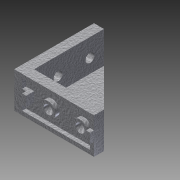
# Autodesk Inventor part: Corner Brace
Saved by Autodesk Inventor 2015 SP1 (Build 190203100, 203)
## iProperties
Created: 2015-03-03
Part Number: Corner Brace
Material: Aluminum 6061
Document SubType Name: Modeling
Designer: Andrew
Density: 2.7 g/cm^3
Appearance: Aluminum Cast
Author: Andrew
Autodesk Inventor part; units mm, degrees
ref_plane "YZ Plane" through (0, 0, 0) normal (1, 0, 0) x (0, 1, 0)
ref_plane "XZ Plane" through (0, 0, 0) normal (0, 1, 0) x (-1, 0, 0)
ref_plane "XY Plane" through (0, 0, 0) normal (0, 0, 1) x (1, 0, 0)
sketch "Sketch1" plane through (0, 0, 0) normal (0, 0, 1) x (1, 0, 0)
  line L0 (0, 0) -> (0, 35)
  line L1 (0, 35) -> (-3, 35)
  line L2 (-3, 35) -> (-3, -3)
  line L3 (-3, -3) -> (35, -3)
  line L4 (35, -3) -> (35, 0)
  line L5 (35, 0) -> (0, 0)
  line L6 (0, 35) -> (35, 0)
  dimension "d0" = 38
  dimension "d1" = 3
  constraints: 14 end point, 7 perpendicular, 1 vertical
  measures "d0" distance between parallel lines of L4 L2
  measures "d1" distance of L0.end L1.end
extrude "Extrusion1" add sketch "Sketch1" along normal blind 18 contours L5 L4 L3 L2 L1 L0
extrude "Extrusion2" add sketch "Sketch1" along normal blind 2 contours L0 L6 L5
sketch "Sketch2" plane through (-3, -3, 0) normal (-1, 0, 0) x (0, 0, 1)
  line L0 (0, 38) -> (0, 0) projected
  line L1 (0, 0) -> (18, 0) projected
  line L2 (18, 38) -> (18, 0) projected
  line L3 (0, 38) -> (18, 38) projected
  line L4 (16, 36) -> (2, 36)
  line L5 (2, 36) -> (2, 2)
  line L6 (2, 2) -> (6.5, 2)
  line L7 (6.5, 2) -> (6.5, 6)
  line L8 (6.5, 6) -> (11.5, 6)
  line L9 (11.5, 6) -> (11.5, 2)
  line L10 (11.5, 2) -> (16, 2)
  line L11 (16, 2) -> (16, 36)
  line L12 (9, 6) -> (9, 0) construction
  line L13 (6.5, 4) -> (11.5, 4)
  line L14 (0, 38) -> (18, 38) projected
  line L15 (6.5, 38) -> (6.5, 36)
  line L16 (11.5, 36) -> (11.5, 38)
  circle A0 centre (9, 31) radius 3.75
  circle A1 centre (9, 15) radius 3.75
  circle A2 centre (9, 31) radius 2.25
  circle A3 centre (9, 15) radius 2.25
  circle A4 centre (9, 31) radius 3
  circle A5 centre (9, 15) radius 3
  line L17 (9, 38) -> (9, 6) construction
  point P0 (0, 3)
  dimension "d6" = 2
  dimension "d7" = 2
  dimension "d8" = 2
  dimension "d9" = 2
  dimension "d10" = 5
  dimension "d11" = 4
  dimension "d12" = 4.5
  dimension "d13" = 0.75
  dimension "d14" = 0.75
  dimension "d15" = 16
  dimension "d16" = 5
  constraints: 26 end point, 8 point on line, 7 perpendicular, 6 centre point, 5 midpoint, 4 coincident, 3 equal radius, 2 collinear, 1 horizontal, 1 parallel, 1 vertical, 1 other
  measures "d6" distance between parallel lines of L0 L5
  measures "d7" distance between parallel lines of L3 L4
  measures "d8" distance between parallel lines of L2 L11
  measures "d9" distance between parallel lines of L1 L6
  measures "d10" distance between parallel lines of L9 L7
  measures "d11" distance between parallel lines of L10 L8
  measures "d12" diameter of A2
  measures "d13" radial gap between concentric circles of A4 A2
  measures "d14" radial gap between concentric circles of A0 A4
  measures "d15" distance of A0.centre A1.centre
  measures "d16" distance from line of L4 A0.centre
extrude "Extrusion3" add sketch "Sketch2" along normal blind 2 contours L3 L15 L4 L5 L6 L7 L13 L9 L10 L11 L16 L2 L1 L0 | L3 L16 L4 L15
extrude "Extrusion4" add sketch "Sketch2" along normal blind 4 contours L3 L16 L4 L15
extrude "Extrusion5" add sketch "Sketch2" along normal blind 4 contours L7 L8 L9 L13
extrude "Extrusion6" add sketch "Sketch2" along normal up to surface (2 mm away) contours A0 | A1 | A4 | A5
extrude "Extrusion7" cut sketch "Sketch2" against normal up to next contours A2 | A3
chamfer "Chamfer1" distance 2 angle 15 1 edges at (-5, 28, 5.25) measured on face at (-4.5, 28, 5.25)
chamfer "Chamfer2" distance 2 angle 15 1 edges at (-5, 12, 5.25) measured on face at (-4.5, 12, 5.25)
sketch "Sketch3" plane through (35, -3, 0) normal (0, -1, 0) x (1, 0, 0)
  line L0 (-2, 16) -> (-2, 2)
  line L1 (-2, 2) -> (-36, 2)
  line L2 (-36, 2) -> (-36, 11.5)
  line L3 (-36, 11.5) -> (-32, 11.5)
  line L4 (-32, 11.5) -> (-32, 6.5)
  line L5 (-32, 6.5) -> (-36, 6.5)
  line L6 (-36, 6.5) -> (-36, 16)
  line L7 (-36, 16) -> (-2, 16)
  line L8 (-32, 9) -> (-40, 9) construction
  line L9 (-34, 11.5) -> (-34, 6.5)
  line L10 (0, 11.5) -> (-2, 11.5)
  line L11 (-2, 6.5) -> (0, 6.5)
  circle A0 centre (-7, 9) radius 3.75
  circle A1 centre (-23, 9) radius 3.75
  circle A2 centre (-7, 9) radius 2.25
  circle A3 centre (-23, 9) radius 2.25
  circle A4 centre (-7, 9) radius 3
  circle A5 centre (-23, 9) radius 3
  line L12 (0, 9) -> (-32, 9) construction
  line L13 (0, 0) -> (-40, 0) projected
  line L14 (0, 0) -> (0, 18) projected
  line L15 (0, 18) -> (-40, 18) projected
  line L16 (-40, 0) -> (-40, 18) projected
  line L17 (0, 0) -> (0, 18) projected
  point P0 (-35, 0)
  point P1 (0, 3)
  dimension "d37" = 5
  dimension "d38" = 4
  dimension "d39" = 4.5
  dimension "d40" = 0.75
  dimension "d41" = 0.75
  dimension "d42" = 16
  dimension "d43" = 5
  dimension "d44" = 2
  dimension "d45" = 4
  dimension "d46" = 2
  constraints: 26 end point, 8 point on line, 6 centre point, 6 perpendicular, 5 midpoint, 4 coincident, 3 collinear, 3 equal radius, 1 parallel, 1 other
  measures "d37" distance between parallel lines of L5 L3
  measures "d38" distance between parallel lines of L6 L4
  measures "d39" diameter of A2
  measures "d40" radial gap between concentric circles of A4 A2
  measures "d41" radial gap between concentric circles of A0 A4
  measures "d42" distance of A0.centre A1.centre
  measures "d43" distance from line of L0 A0.centre
  measures "d44" distance between parallel lines of L13 L1
  measures "d45" distance between parallel lines of L16 L2
  measures "d46" distance between parallel lines of L14 L0
extrude "Extrusion8" add sketch "Sketch3" along normal blind 2 contours L7 L6 L2 L1 L0 L11 L14 L13 L16 L15 L10 | L3 L9 L5 L2 | A0 | A1 | A4 | A5
extrude "Extrusion9" add sketch "Sketch3" along normal blind 4 contours L10 L14 L11 L0 | L3 L4 L5 L9
extrude "Extrusion10" cut sketch "Sketch3" against normal up to next contours A2 | A3
body "Solid1"
